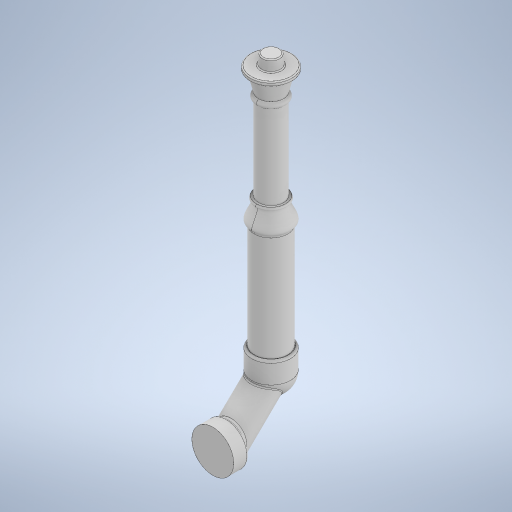
# Autodesk Inventor part: 塔2
Saved by Autodesk Inventor 2024 (Build 280153000, 153)
## iProperties
Created: 2024-05-25
Part Number: 塔2
Material: 一般
Document SubType Name: Modeling
Designer: User
Density: 1 g/cm^3
Appearance: 預設
Author: User
Autodesk Inventor part; units mm, degrees
ref_plane "YZ Plane" through (0, 0, 0) normal (1, 0, 0) x (0, 1, 0)
ref_plane "XY Plane" through (0, 0, 0) normal (0, 0, 1) x (1, 0, 0)
sketch "草圖1" plane through (0, 0, 0) normal (0, 0, 1) x (1, 0, 0)
  circle A0 centre (0, 0) radius 10
  circle A1 centre (0, 0) radius 8
  dimension "d0" = 20
  dimension "d1" = 16
  constraints: 2 centre point, 2 coincident
  measures "d0" diameter of A0
  measures "d1" diameter of A1
extrude "擠出1" add sketch "草圖1" along normal blind 7.3
extrude "擠出2" add sketch "草圖1" along normal blind 7.3 contours A1
sketch "草圖2" plane through (0, 0, 0) normal (0, 0, -1) x (-1, 0, 0)
  circle A0 centre (0, 0) radius 8
  dimension "d6" = 16
  constraints: 1 centre point, 1 coincident
  measures "d6" diameter of A0
ref_plane "工作平面1" through (0, 20, 0) normal (0, 1, 0) x (-1, 0, 0)
sketch "草圖3" plane through (0, 20, 0) normal (0, 1, 0) x (-1, 0, 0)
  circle A0 centre (0, -20.5453) radius 8
  point P0 (0, 0)
  dimension "d8" = 16
  constraints: 1 centre point
  measures "d8" diameter of A0
loft "斷面混成1" add profiles "草圖3", "草圖2"
sketch "草圖4" plane through (0, 20, -20.5453) normal (0, 1, 0) x (1, 0, 0)
  circle A0 centre (0, 0) radius 9.25
  line L0 (9.25, 0) -> (-9.4837, 0)
  line L1 (-8, 0) -> (-8, -20.5453) projected
  point P0 (0, -20.5453)
  point P1 (-9.25, 0)
  dimension "d13" = 18.5
  constraints: 2 end point, 1 perpendicular, 3 other
revolve "迴轉1" add sketch "草圖4" angle 180 about axis through (9.25, 20, -20.5453) along (-1, 0, 0) contours L0 A0
sketch "草圖5" plane through (0, 20, -20.5453) normal (0, 1, 0) x (1, 0, 0)
  circle A0 centre (0, 0) radius 9.25
  circle A1 centre (0, 0) radius 9.25 projected
  point P0 (0, -20.5453)
  constraints: 1 centre point, 1 concentric
extrude "擠出3" add sketch "草圖5" along normal blind 10
sketch "草圖6" plane through (0, 30, -20.5453) normal (0, 1, 0) x (1, 0, 0)
  circle A0 centre (0, 0) radius 8
  point P0 (0, -20.5453)
  dimension "d17" = 16
  constraints: 1 centre point
  measures "d17" diameter of A0
extrude "擠出4" add sketch "草圖6" along normal blind 50
fillet "圓角1" radius 1 4 edges at (-9.25, 30, -20.5453) (8, 16.7517, -17.227) (-10, 0, 0) (8, 0, 0)
sketch "草圖7" plane through (0, 0, 0) normal (1, 0, 0) x (0, 1, 0)
  line L0 (80, -28.5453) -> (80, -12.5453) projected
  line L1 (80, -20.5453) -> (92, -20.5453)
  line L2 (92, -20.5453) -> (92, -13.5453)
  spline S0 degree 4 poles (92, -13.5453) (89.365, -12.032) (94.8705, -19.0296) (78.4645, -7.0884) (82.4871, -12.5131) (80, -12.5453) knots 0 0 0 0 0 0.467099 1 1 1 1 1
  line L3 (80, -20.5453) -> (80, -12.5453)
  point P0 (0, 0)
  point P1 (90.6563, -13.5453)
  point P2 (90.2228, -14.1558)
  point P3 (83.6337, -11.5548)
  point P4 (81.5962, -11.5548)
  dimension "d21" = 12
  dimension "d22" = 7
  constraints: 6 end point, 1 collinear, 1 horizontal, 1 midpoint, 1 perpendicular, 6 other
  measures "d21" distance of L1.start L1.end
  measures "d22" distance of L1.end L2.end
revolve "迴轉2" add sketch "草圖7" angle 360 about axis through (0, 80, -20.5453) along (0, 1, 0)
sketch "草圖8" plane through (0, 92, -20.5453) normal (0, 1, 0) x (1, 0, 0)
  circle A0 centre (0, 0) radius 8 projected
  circle A1 centre (0, 0) radius 6
  point P0 (0, -20.5453)
  dimension "d24" = 12
  constraints: 1 centre point, 1 coincident
  measures "d24" diameter of A1
extrude "擠出5" add sketch "草圖8" along normal blind 40 contours A1
sketch "草圖9" plane through (0, 0, 0) normal (1, 0, 0) x (0, 1, 0)
  line L0 (132, -26.5453) -> (132, -14.5453) projected
  line L1 (132, -20.5453) -> (146, -20.5453)
  line L2 (146, -20.5453) -> (146, -11.0453)
  line L3 (145.5, -10.5453) -> (144.4015, -10.5453)
  line L4 (143.9133, -10.9373) -> (143.6357, -12.1925)
  line L5 (143.2637, -12.5708) -> (134.9989, -14.5453)
  spline S0 degree 2 poles (134.9989, -14.5453) (133.2452, -12.5001) (132, -14.5453) knots 0 0 0 1 1 1
  arc A0 (146, -11.0453) -> (145.5, -10.5453) centre (145.5, -11.0453) ccw
  arc A1 (144.4015, -10.5453) -> (143.9133, -10.9373) centre (144.4015, -11.0453) ccw
  arc A2 (143.2637, -12.5708) -> (143.6357, -12.1925) centre (143.1475, -12.0845) ccw
  point P0 (0, 0)
  point P1 (146, -10.5453)
  point P2 (144, -10.5453)
  point P3 (143.5681, -12.4981)
  point P4 (133.3069, -13.5247)
  dimension "d27" = 14
  dimension "d28" = 10
  dimension "d29" = 2
  dimension "d30" = 2
  dimension "d31" = 0.5
  constraints: 10 end point, 6 point on circle, 6 point on line, 6 tangent, 3 centre point, 2 equal radius, 2 horizontal, 1 midpoint, 1 vertical, 3 other
  measures "d27" distance of L1.start L1.end
  measures "d28" distance of L1.end point (146, -10.545)
  measures "d29" distance of point (146, -10.545) point (144, -10.545)
  measures "d30" distance of point (144, -10.545) point (143.568, -12.498)
  measures "d31" radius of A0
revolve "迴轉3" add sketch "草圖9" angle 360 about axis through (0, 132, -20.5453) along (0, 1, 0)
sketch "草圖10" plane through (0, 146, -20.5453) normal (0, 1, 0) x (1, 0, 0)
  circle A0 centre (0, 0) radius 6 projected
  circle A1 centre (0, 0) radius 4.5
  point P0 (0, -20.5453)
  dimension "d33" = 9
  constraints: 1 centre point, 1 coincident
  measures "d33" diameter of A1
extrude "擠出6" add sketch "草圖10" along normal blind 5 draft -5 contours A1
fillet "圓角2" radius 0.5 1 edges at (-4.0626, 151, -20.5453)
fillet "圓角3" radius 0.5 1 edges at (-4.5, 146, -20.5453)
